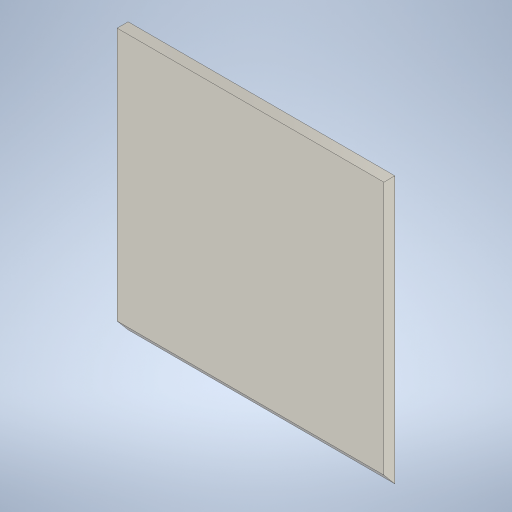
# Autodesk Inventor part: MetalBottom
Saved by Autodesk Inventor 2023 (Build 270158000, 158)
## iProperties
Created: 2024-03-04
Part Number: MetalBottom
Material: Generic
Document SubType Name: Modeling
Designer: pavel
Density: 1 g/cm^3
Appearance: Default
Author: pavel
Autodesk Inventor part; units mm, degrees
ref_plane "YZ Plane" through (0, 0, 0) normal (1, 0, 0) x (0, 1, 0)
ref_plane "XZ Plane" through (0, 0, 0) normal (0, 1, 0) x (-1, 0, 0)
ref_plane "XY Plane" through (0, 0, 0) normal (0, 0, 1) x (1, 0, 0)
sketch "Sketch1" plane through (0, 0, 0) normal (0, 0, 1) x (1, 0, 0)
  line L0 (0, 0) -> (97, 0)
  line L1 (97, 0) -> (97, 97)
  line L2 (97, 97) -> (0, 97)
  line L3 (0, 97) -> (0, 0)
  dimension "d0" = 97
  dimension "d1" = 97
  constraints: 8 end point, 2 parallel, 1 horizontal, 1 perpendicular
  measures "d0" distance of L2.end L1.end
  measures "d1" distance of L1.end L0.end
extrude "Extrusion1" add sketch "Sketch1" along normal blind 4
sketch "Sketch3" plane through (97, 0, 0) normal (1, 0, 0) x (0, 0, -1)
  line L0 (0, 0) -> (-4, 0) projected
  line L1 (0, 0) -> (-11, 13.1093)
  line L2 (0, 0) -> (0, 97) projected
  line L3 (0, 97) -> (-4, 97) projected
  line L4 (-4, 0) -> (-4, 97) projected
  line L5 (0, 0) -> (-4, 0) projected
  point P0 (-4, 4.767)
  dimension "d11" = 7
  dimension "d12" = 40
  constraints: 2 end point
  measures "d11" distance from line of L4 L1.end
  measures "d12" angle of L2 L1
extrude "Extrusion2" cut sketch "Sketch3" against normal through all contours L0 L4 L1
body "Solid1"
